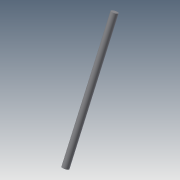
# Autodesk Inventor part: Carriage Tooth
Saved by Autodesk Inventor 2014 SP1 (Build 180222100, 222)
## iProperties
Created: 2014-03-26
Part Number: Carriage Tooth
Material: Generic
Document SubType Name: Modeling
Designer: tom
Density: 1 g/cm^3
Appearance: Default
Author: tom
Autodesk Inventor part; units mm, degrees
ref_plane "YZ Plane" through (0, 0, 0) normal (1, 0, 0) x (0, 1, 0)
ref_plane "XZ Plane" through (0, 0, 0) normal (0, 1, 0) x (-1, 0, 0)
ref_plane "XY Plane" through (0, 0, 0) normal (0, 0, 1) x (1, 0, 0)
sketch "Sketch1" plane through (0, 0, 0) normal (1, 0, 0) x (0, 1, 0)
  spline S0 degree 3 poles (-4.479, -27.0431) (-4.7662, -26.7746) (-5.439, -26.5061) (-6.0629, -26.2376) (-6.6869, -25.9691) (-7.2127, -25.7006) (-7.3009, -25.4322) (-7.389, -25.1637) (-7.0326, -24.8952) (-6.4617, -24.6267) (-5.8908, -24.3582) (-5.1506, -24.0897) (-4.7189, -23.8212) (-4.2873, -23.5527) (-4.1983, -23.2842) (-4.5096, -23.0157) (-4.8208, -22.7472) (-5.5075, -22.4787) (-6.1264, -22.2102) (-6.7453, -21.9417) (-7.2474, -21.6732) (-7.3085, -21.4047) (-7.3696, -21.1362) (-6.9849, -20.8677) (-6.4028, -20.5992) (-5.8207, -20.3307) (-5.0872, -20.0622) (-4.6758, -19.7937) (-4.2645, -19.5252) (-4.2079, -19.2568) (-4.5426, -18.9883) (-4.8772, -18.7198) (-5.5767, -18.4513) (-6.1893, -18.1828) (-6.802, -17.9143) (-7.2794, -17.6458) (-7.3133, -17.3773) (-7.3473, -17.1088) (-6.935, -16.8403) (-6.3428, -16.5718) (-5.7505, -16.3033) (-5.0251, -16.0348) (-4.6349, -15.7663) (-4.2446, -15.4978) (-4.2205, -15.2293) (-4.5779, -14.9608) (-4.9354, -14.6923) (-5.6463, -14.4238) (-6.2516, -14.1553) (-6.8569, -13.8868) (-7.3087, -13.6183) (-7.3154, -13.3498) (-7.3221, -13.0814) (-6.8831, -12.8129) (-6.2818, -12.5444) (-5.6805, -12.2759) (-4.9645, -12.0074) (-4.5961, -11.7389) (-4.2277, -11.4704) (-4.236, -11.2019) (-4.6156, -10.9334) (-4.9952, -10.6649) (-5.7162, -10.3964) (-6.313, -10.1279) (-6.9098, -9.8594) (-7.3353, -9.5909) (-7.3147, -9.3224) (-7.2941, -9.0539) (-6.8291, -8.7854) (-6.22, -8.5169) (-5.6108, -8.2484) (-4.9055, -7.9799) (-4.5596, -7.7114) (-4.2137, -7.4429) (-4.2544, -7.1745) (-4.6555, -6.906) (-5.0566, -6.6375) (-5.7863, -6.369) (-6.3735, -6.1005) (-6.9607, -5.832) (-7.359, -5.5635) (-7.3112, -5.295) (-7.2634, -5.0265) (-6.7733, -4.758) (-6.1573, -4.4895) (-5.5414, -4.221) (-4.8482, -3.9525) (-4.5255, -3.684) (-4.2027, -3.4155) (-4.2758, -3.147) (-4.6975, -2.8785) (-5.1193, -2.61) (-5.8564, -2.3415) (-6.433, -2.073) (-7.0095, -1.8045) (-7.3799, -1.536) (-7.3049, -1.2675) (-7.23, -0.9991) (-6.7157, -0.7306) (-6.0941, -0.4621) (-5.4725, -0.1936) (-4.7927, 0.0749) (-4.4937, 0.3434) (-4.1946, 0.6119) (-4.3, 0.8804) (-4.7417, 1.1489) (-5.1834, 1.4174) (-5.9265, 1.6859) (-6.4913, 1.9544) (-7.0561, 2.2229) (-7.3978, 2.4914) (-7.2959, 2.7599) (-7.194, 3.0284) (-6.6565, 3.2969) (-6.0304, 3.5654) (-5.4043, 3.8339) (-4.7391, 4.1024) (-4.4644, 4.3709) (-4.1896, 4.6394) (-4.327, 4.9079) (-4.7878, 5.1763) (-5.2486, 5.4448) (-5.9964, 5.7133) (-6.5483, 5.9818) (-7.1003, 6.2503) (-7.4128, 6.5188) (-7.2841, 6.7873) (-7.1554, 7.0558) (-6.5956, 7.3243) (-5.9662, 7.5928) (-5.3368, 7.8613) (-4.6875, 8.1298) (-4.4375, 8.3983) (-4.1876, 8.6668) (-4.3567, 8.9353) (-4.8358, 9.2038) (-5.3148, 9.4723) (-6.0659, 9.7408) (-6.604, 10.0093) (-7.1422, 10.2778) (-7.4249, 10.5463) (-7.2696, 10.8148) (-7.1143, 11.0832) (-6.5334, 11.3517) (-5.9018, 11.6202) (-5.2702, 11.8887) (-4.638, 12.1572) (-4.4133, 12.4257) (-4.1886, 12.6942) (-4.3892, 12.9627) (-4.8856, 13.2312) (-5.382, 13.4997) (-6.135, 13.7682) (-6.6583, 14.0367) (-7.1816, 14.3052) (-7.434, 14.5737) (-7.2524, 14.8422) (-7.0708, 15.1107) (-6.4697, 15.3792) (-5.8372, 15.6477) (-5.2046, 15.9162) (-4.5906, 16.1847) (-4.3916, 16.4532) (-4.1926, 16.7217) (-4.4244, 16.9902) (-4.9372, 17.2586) (-5.45, 17.5271) (-6.2034, 17.7956) (-6.711, 18.0641) (-7.2185, 18.3326) (-7.44, 18.6011) (-7.2325, 18.8696) (-7.025, 19.1381) (-6.4049, 19.4066) (-5.7725, 19.6751) (-5.1402, 19.9436) (-4.5456, 20.2121) (-4.3726, 20.4806) (-4.1997, 20.7491) (-4.4621, 21.0176) (-4.9904, 21.2861) (-5.5187, 21.5546) (-6.2712, 21.8231) (-6.762, 22.0916) (-7.2528, 22.3601) (-7.4431, 22.6286) (-7.21, 22.8971) (-6.977, 23.1656) (-6.339, 23.434) (-5.708, 23.7025) (-5.077, 23.971) (-4.5029, 24.2395) (-4.3563, 24.508) (-4.3292, 24.5576) (-4.3155, 24.6073) (-4.3155, 24.6569) knots -81.21017 -81.21017 -81.21017 -81.21017 -79.944914 -79.944914 -79.944914 -78.679659 -78.679659 -78.679659 -77.414403 -77.414403 -77.414403 -76.149147 -76.149147 -76.149147 -74.883892 -74.883892 -74.883892 -73.618636 -73.618636 -73.618636 -72.35338 -72.35338 -72.35338 -71.088125 -71.088125 -71.088125 -69.822869 -69.822869 -69.822869 -68.557613 -68.557613 -68.557613 -67.292358 -67.292358 -67.292358 -66.027102 -66.027102 -66.027102 -64.761846 -64.761846 -64.761846 -63.496591 -63.496591 -63.496591 -62.231335 -62.231335 -62.231335 -60.96608 -60.96608 -60.96608 -59.700824 -59.700824 -59.700824 -58.435568 -58.435568 -58.435568 -57.170313 -57.170313 -57.170313 -55.905057 -55.905057 -55.905057 -54.639801 -54.639801 -54.639801 -53.374546 -53.374546 -53.374546 -52.10929 -52.10929 -52.10929 -50.844034 -50.844034 -50.844034 -49.578779 -49.578779 -49.578779 -48.313523 -48.313523 -48.313523 -47.048267 -47.048267 -47.048267 -45.783012 -45.783012 -45.783012 -44.517756 -44.517756 -44.517756 -43.2525 -43.2525 -43.2525 -41.987245 -41.987245 -41.987245 -40.721989 -40.721989 -40.721989 -39.456733 -39.456733 -39.456733 -38.191478 -38.191478 -38.191478 -36.926222 -36.926222 -36.926222 -35.660966 -35.660966 -35.660966 -34.395711 -34.395711 -34.395711 -33.130455 -33.130455 -33.130455 -31.865199 -31.865199 -31.865199 -30.599944 -30.599944 -30.599944 -29.334688 -29.334688 -29.334688 -28.069432 -28.069432 -28.069432 -26.804177 -26.804177 -26.804177 -25.538921 -25.538921 -25.538921 -24.273665 -24.273665 -24.273665 -23.00841 -23.00841 -23.00841 -21.743154 -21.743154 -21.743154 -20.477898 -20.477898 -20.477898 -19.212643 -19.212643 -19.212643 -17.947387 -17.947387 -17.947387 -16.682131 -16.682131 -16.682131 -15.416876 -15.416876 -15.416876 -14.15162 -14.15162 -14.15162 -12.886364 -12.886364 -12.886364 -11.621109 -11.621109 -11.621109 -10.355853 -10.355853 -10.355853 -9.090597 -9.090597 -9.090597 -7.825342 -7.825342 -7.825342 -6.560086 -6.560086 -6.560086 -5.29483 -5.29483 -5.29483 -4.029575 -4.029575 -4.029575 -2.764319 -2.764319 -2.764319 -1.499063 -1.499063 -1.499063 -0.233808 -0.233808 -0.233808 0 0 0 0 projected
  spline S1 degree 3 poles (-4.3155, 25.6569) (-4.3155, 25.3884) (-4.761, 25.1199) (-5.3643, 24.8514) (-5.9676, 24.5829) (-6.6811, 24.3144) (-7.044, 24.0459) (-7.407, 23.7774) (-7.3908, 23.5089) (-7.0058, 23.2404) (-6.6209, 22.9719) (-5.8977, 22.7034) (-5.3031, 22.4349) (-4.7085, 22.1664) (-4.2896, 21.8979) (-4.3169, 21.6294) (-4.3441, 21.3609) (-4.8154, 21.0925) (-5.4263, 20.824) (-6.0373, 20.5555) (-6.7397, 20.287) (-7.08, 20.0185) (-7.4203, 19.75) (-7.3716, 19.4815) (-6.9654, 19.213) (-6.5592, 18.9445) (-5.8275, 18.676) (-5.2428, 18.4075) (-4.6581, 18.139) (-4.2666, 17.8705) (-4.3211, 17.602) (-4.3755, 17.3335) (-4.8716, 17.065) (-5.4891, 16.7965) (-6.1066, 16.528) (-6.7965, 16.2595) (-7.1136, 15.991) (-7.4306, 15.7225) (-7.3496, 15.454) (-6.9228, 15.1855) (-6.4961, 14.9171) (-5.7574, 14.6486) (-5.1836, 14.3801) (-4.6099, 14.1116) (-4.2465, 13.8431) (-4.328, 13.5746) (-4.4096, 13.3061) (-4.9297, 13.0376) (-5.5525, 12.7691) (-6.1753, 12.5006) (-6.8516, 12.2321) (-7.1447, 11.9636) (-7.4379, 11.6951) (-7.3247, 11.4266) (-6.8782, 11.1581) (-6.4318, 10.8896) (-5.6874, 10.6211) (-5.1256, 10.3526) (-4.5639, 10.0841) (-4.2292, 9.8156) (-4.3377, 9.5471) (-4.4462, 9.2786) (-4.9893, 9.0101) (-5.6163, 8.7417) (-6.2434, 8.4732) (-6.9047, 8.2047) (-7.1735, 7.9362) (-7.4422, 7.6677) (-7.297, 7.3992) (-6.8316, 7.1307) (-6.3663, 6.8622) (-5.6176, 6.5937) (-5.0689, 6.3252) (-4.5202, 6.0567) (-4.2149, 5.7882) (-4.3502, 5.5197) (-4.4854, 5.2512) (-5.0505, 4.9827) (-5.6806, 4.7142) (-6.3106, 4.4457) (-6.9558, 4.1772) (-7.1996, 3.9087) (-7.4434, 3.6402) (-7.2665, 3.3717) (-6.7832, 3.1032) (-6.2998, 2.8348) (-5.5481, 2.5663) (-5.0135, 2.2978) (-4.4789, 2.0293) (-4.2036, 1.7608) (-4.3654, 1.4923) (-4.5271, 1.2238) (-5.1131, 0.9553) (-5.7451, 0.6868) (-6.377, 0.4183) (-7.0048, 0.1498) (-7.2233, -0.1187) (-7.4417, -0.3872) (-7.2334, -0.6557) (-6.7329, -0.9242) (-6.2324, -1.1927) (-5.4792, -1.4612) (-4.9597, -1.7297) (-4.4401, -1.9982) (-4.1953, -2.2667) (-4.3832, -2.5352) (-4.5712, -2.8037) (-5.177, -3.0722) (-5.8097, -3.3406) (-6.4423, -3.6091) (-7.0516, -3.8776) (-7.2443, -4.1461) (-7.4369, -4.4146) (-7.1976, -4.6831) (-6.6809, -4.9516) (-6.1642, -5.2201) (-5.4109, -5.4886) (-4.9074, -5.7571) (-4.4039, -6.0256) (-4.19, -6.2941) (-4.4038, -6.5626) (-4.6176, -6.8311) (-5.2422, -7.0996) (-5.8743, -7.3681) (-6.5064, -7.6366) (-7.0961, -7.9051) (-7.2626, -8.1736) (-7.4291, -8.4421) (-7.1593, -8.7106) (-6.6273, -8.9791) (-6.0954, -9.2476) (-5.3433, -9.516) (-4.8568, -9.7845) (-4.3702, -10.053) (-4.1877, -10.3215) (-4.4269, -10.59) (-4.6662, -10.8585) (-5.3083, -11.127) (-5.9388, -11.3955) (-6.5693, -11.664) (-7.1382, -11.9325) (-7.2783, -12.201) (-7.4183, -12.4695) (-7.1185, -12.738) (-6.5722, -13.0065) (-6.026, -13.275) (-5.2767, -13.5435) (-4.808, -13.812) (-4.3393, -14.0805) (-4.1884, -14.349) (-4.4526, -14.6175) (-4.7169, -14.886) (-5.3754, -15.1545) (-6.0031, -15.4229) (-6.6308, -15.6914) (-7.1779, -15.9599) (-7.2912, -16.2284) (-7.4046, -16.4969) (-7.0752, -16.7654) (-6.5157, -17.0339) (-5.9563, -17.3024) (-5.211, -17.5709) (-4.761, -17.8394) (-4.3111, -18.1079) (-4.1921, -18.3764) (-4.4809, -18.6449) (-4.7697, -18.9134) (-5.4434, -19.1819) (-6.067, -19.4504) (-6.6907, -19.7189) (-7.215, -19.9874) (-7.3014, -20.2559) (-7.3879, -20.5244) (-7.0296, -20.7929) (-6.4579, -21.0614) (-5.8863, -21.3299) (-5.1464, -21.5983) (-4.7161, -21.8668) (-4.2857, -22.1353) (-4.1989, -22.4038) (-4.5116, -22.6723) (-4.8244, -22.9408) (-5.512, -23.2093) (-6.1305, -23.4778) (-6.749, -23.7463) (-7.2495, -24.0148) (-7.3089, -24.2833) (-7.3682, -24.5518) (-6.9818, -24.8203) (-6.3989, -25.0888) (-5.8161, -25.3573) (-5.0831, -25.6258) (-4.6731, -25.8943) (-4.2631, -26.1628) (-4.2086, -26.4313) (-4.5448, -26.6998) (-4.6881, -26.8142) (-4.8942, -26.9287) (-5.1345, -27.0431) knots 0 0 0 0 1.265256 1.265256 1.265256 2.530511 2.530511 2.530511 3.795767 3.795767 3.795767 5.061023 5.061023 5.061023 6.326278 6.326278 6.326278 7.591534 7.591534 7.591534 8.85679 8.85679 8.85679 10.122045 10.122045 10.122045 11.387301 11.387301 11.387301 12.652557 12.652557 12.652557 13.917812 13.917812 13.917812 15.183068 15.183068 15.183068 16.448324 16.448324 16.448324 17.713579 17.713579 17.713579 18.978835 18.978835 18.978835 20.244091 20.244091 20.244091 21.509346 21.509346 21.509346 22.774602 22.774602 22.774602 24.039858 24.039858 24.039858 25.305113 25.305113 25.305113 26.570369 26.570369 26.570369 27.835625 27.835625 27.835625 29.10088 29.10088 29.10088 30.366136 30.366136 30.366136 31.631392 31.631392 31.631392 32.896647 32.896647 32.896647 34.161903 34.161903 34.161903 35.427159 35.427159 35.427159 36.692414 36.692414 36.692414 37.95767 37.95767 37.95767 39.222926 39.222926 39.222926 40.488181 40.488181 40.488181 41.753437 41.753437 41.753437 43.018693 43.018693 43.018693 44.283948 44.283948 44.283948 45.549204 45.549204 45.549204 46.814459 46.814459 46.814459 48.079715 48.079715 48.079715 49.344971 49.344971 49.344971 50.610226 50.610226 50.610226 51.875482 51.875482 51.875482 53.140738 53.140738 53.140738 54.405993 54.405993 54.405993 55.671249 55.671249 55.671249 56.936505 56.936505 56.936505 58.20176 58.20176 58.20176 59.467016 59.467016 59.467016 60.732272 60.732272 60.732272 61.997527 61.997527 61.997527 63.262783 63.262783 63.262783 64.528039 64.528039 64.528039 65.793294 65.793294 65.793294 67.05855 67.05855 67.05855 68.323806 68.323806 68.323806 69.589061 69.589061 69.589061 70.854317 70.854317 70.854317 72.119573 72.119573 72.119573 73.384828 73.384828 73.384828 74.650084 74.650084 74.650084 75.91534 75.91534 75.91534 77.180595 77.180595 77.180595 78.445851 78.445851 78.445851 79.711107 79.711107 79.711107 80.976362 80.976362 80.976362 82.241618 82.241618 82.241618 82.780966 82.780966 82.780966 82.780966 projected
  line L0 (-4.7597, 6.1899) -> (4.004, 2.288)
  line L1 (-5.1314, 6.3554) -> (4.8686, 6.3554) construction
  line L2 (-5.1314, 5.355) -> (3.6323, 1.4531)
  line L3 (-5.1314, 5.355) -> (4.8686, 5.355) construction
  line L4 (4.004, 2.288) -> (3.6323, 1.4531)
  line L5 (-5.1314, 5.355) -> (-4.7597, 6.1899)
  point P0 (0, 0)
  dimension "d1" = 24
  dimension "d3" = 24
  constraints: 12 end point, 2 horizontal, 2 perpendicular, 1 parallel, 2 other
  measures "d1" angle of L0 L1
  measures "d3" angle of L2 L3
extrude "Extrusion1" add sketch "Sketch1" along normal blind 0.914 contours L5 S1 L2 | S1 L5 L0 L4 L2
sketch "Sketch2" plane through (0, 4.004, 2.288) normal (0, 0.9135455, -0.4067366) x (1, 0, 0)
  line L0 (0, 0.9139) -> (0, 0) projected
  line L1 (0, 0) -> (0.914, 0) projected
  line L2 (0.914, 0.9139) -> (0.914, 0) projected
  line L3 (0, 0.9139) -> (0.914, 0.9139) projected
  line L4 (0.457, 0.9139) -> (0.457, 0) construction
  line L5 (0.914, 0.457) -> (0, 0.457) construction
  circle A0 centre (0.457, 0.457) radius 0.457
  constraints: 5 midpoint, 4 end point, 1 vertical alignment, 2 other
extrude "Extrusion2" cut sketch "Sketch2" against normal blind 20 contours L3 A0 L0 | A0 L1 L0 | L3 L2 A0 | A0 L2 L1
sketch "Sketch3" plane through (0.457, 3.8182, 1.8706) normal (0, 0.9135455, -0.4067366) x (1, 0, 0)
  circle A0 centre (0, 0) radius 0.457 projected
  circle A1 centre (0, 0) radius 0.457
  point P0 (-0.457, 3.2618)
  constraints: 1 centre point, 1 coincident, 1 concentric
extrude "Extrusion3" add sketch "Sketch3" along normal blind 8.75
body "Solid1"
